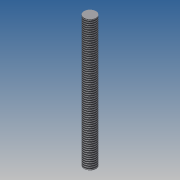
# Autodesk Inventor part: Gewindestück_M5_Z-Achse_55mm
Saved by Autodesk Inventor 2015 SP1 (Build 190203100, 203)
## iProperties
Created: 2015-03-05
Part Number: Gewindestück_M5_Z-Achse_55mm
Material: Generisch
Document SubType Name: Modeling
Designer: Marc
Density: 1 g/cm^3
Appearance: Vorgabe
Author: Marc
Autodesk Inventor part; units mm, degrees
ref_plane "YZ Plane" through (0, 0, 0) normal (1, 0, 0) x (0, 1, 0)
ref_plane "XZ Plane" through (0, 0, 0) normal (0, 1, 0) x (-1, 0, 0)
ref_plane "XY Plane" through (0, 0, 0) normal (0, 0, 1) x (1, 0, 0)
sketch "Skizze1" plane through (0, 0, 0) normal (0, 0, 1) x (1, 0, 0)
  line L0 (-3.5, 0) -> (3.5, 0) projected
  line L1 (0, -3.5) -> (0, 3.5) projected
  circle A0 centre (0, 0) radius 2.5
  dimension "d0" = 5
  constraints: 1 centre point, 1 coincident
  measures "d0" diameter of A0
extrude "Extrusion1" add sketch "Skizze1" along normal mid plane 55
thread "Gewinde1" size "M5x0.8" class "6g" standard "ANSI Metric M Profile" full length
